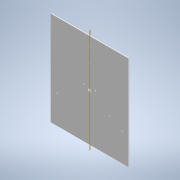
# Autodesk Inventor part: верхняя пластина
Saved by Autodesk Inventor 2021.1 (Build 251245010, 245A)
## iProperties
Created: 2023-01-21
Part Number: верхняя пластина
Material: Типовые
Document SubType Name: Modeling
Designer: zmoze
Density: 1 g/cm^3
Appearance: По умолчанию
Author: zmoze
Autodesk Inventor part; units mm, degrees
ref_plane "XZ Plane" through (0, 0, 0) normal (0, 1, 0) x (-1, 0, 0)
ref_plane "XY Plane" through (0, 0, 0) normal (0, 0, 1) x (1, 0, 0)
sketch "Эскиз1" plane through (0, 0, 0) normal (0, 0, 1) x (1, 0, 0)
  line L0 (-120, 145) -> (120, 145)
  line L1 (120, 145) -> (120, -145)
  line L2 (120, -145) -> (-120, -145)
  line L3 (-120, -145) -> (-120, 145)
  line L4 (-120, 145) -> (120, -145) construction
  line L5 (120, 145) -> (-120, -145) construction
  point P0 (0, 0)
  dimension "d0" = 240
  dimension "d1" = 290
  constraints: 12 end point, 2 midpoint, 2 parallel, 1 horizontal, 1 perpendicular
  measures "d0" distance of L0.start L0.end
  measures "d1" distance of L0.end L1.end
extrude "Выдавливание1" add sketch "Эскиз1" along normal blind 3
sketch "Эскиз2" plane through (0, 0, 3) normal (0, 0, 1) x (1, 0, 0)
  line L0 (-5, 120) -> (5, 120)
  line L1 (120, 145) -> (-120, 145) projected
  line L2 (0, 203) -> (0, -203) projected
  line L3 (-101.423, -64.3301) -> (-106.423, -55.6699)
  line L4 (106.423, -55.6699) -> (101.423, -64.3301)
  point P0 (0, 0)
  point P1 (0, 120)
  point P2 (0, 0)
  point P3 (-103.923, -60)
  point P4 (103.923, -60)
  dimension "d4" = 25
  dimension "d5" = 10
  dimension "d8" = 360
  dimension "d10" = 120
  constraints: 6 end point, 2 midpoint, 1 horizontal, 1 point on line, 13 other
  measures "d4" distance between parallel lines of L0 L1
  measures "d5" distance of L0.start L0.end
  measures "d10" distance from line of point (0, 0) L0
sketch "Эскиз3" plane through (0, 0, 0) normal (0, 0, -1) x (-1, 0, 0)
  circle A0 centre (17.5, 8) radius 2 projected
  circle A1 centre (-17.5, 8) radius 2 projected
  circle A2 centre (-100.892, -58.25) radius 1.5 projected
  circle A3 centre (-62.7868, -36.25) radius 1.5 projected
  circle A4 centre (100.892, -58.25) radius 1.5 projected
  circle A5 centre (62.7868, -36.25) radius 1.5 projected
  circle A6 centre (0, 116.5) radius 1.5 projected
  circle A7 centre (0, 72.5) radius 1.5 projected
  circle A8 centre (0, 0) radius 4.6 projected
  circle A9 centre (0, 0) radius 4.65
  point P0 (0, 0)
  dimension "d13" = 0.05
  constraints: 1 centre point
  measures "d13" radial gap between concentric circles of A9 A8
extrude "Выдавливание2" cut sketch "Эскиз3" against normal through all contours A0 | A1 | A2 | A3 | A4 | A6 | A7 | A8 | A9
